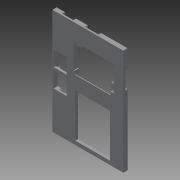
# Autodesk Inventor part: DisplayTop
Saved by Autodesk Inventor 2014 SP1 (Build 180222100, 222)
## iProperties
Created: 2014-03-24
Part Number: DisplayTop
Material: Generic
Document SubType Name: Modeling
Designer: patrigg
Density: 1 g/cm^3
Appearance: Default
Author: patrigg
Autodesk Inventor part; units mm, degrees
ref_plane "YZ Plane" through (0, 0, 0) normal (1, 0, 0) x (0, 1, 0)
ref_plane "XZ Plane" through (0, 0, 0) normal (0, 1, 0) x (-1, 0, 0)
ref_plane "XY Plane" through (0, 0, 0) normal (0, 0, 1) x (1, 0, 0)
sketch "Sketch2" plane through (0, 0, 0) normal (0, 1, 0) x (-1, 0, 0)
  line L0 (-33.5, -50) -> (33.5, -50)
  line L1 (33.5, -50) -> (33.5, 50)
  line L2 (33.5, 50) -> (-33.5, 50)
  line L3 (-33.5, 50) -> (-33.5, -50)
  line L4 (-33.5, -50) -> (33.5, 50) construction
  line L5 (33.5, -50) -> (-33.5, 50) construction
  point P0 (0, 0)
  dimension "d0" = 67
  dimension "d1" = 100
  constraints: 12 end point, 2 midpoint, 2 parallel, 1 horizontal, 1 perpendicular
  measures "d0" distance of L2.end L1.end
  measures "d1" distance of L1.end L0.end
extrude "Extrusion1" add sketch "Sketch2" along normal blind 4
sketch "Sketch3" plane through (0, 4, 0) normal (0, 1, 0) x (1, 0, 0)
  line L0 (33.5, 50) -> (-33.5, 50) projected
  line L1 (-14.5, -4.5) -> (23.5, -4.5)
  line L2 (23.5, -4.5) -> (23.5, 48)
  line L3 (23.5, 48) -> (-14.5, 48)
  line L4 (-14.5, 48) -> (-14.5, -4.5)
  line L5 (-14.5, -4.5) -> (23.5, 48) construction
  line L6 (23.5, -4.5) -> (-14.5, 48) construction
  line L7 (33.5, -50) -> (33.5, 50) projected
  point P0 (0, 0)
  point P1 (4.5, 21.75)
  dimension "d4" = 38
  dimension "d5" = 52.5
  dimension "d6" = 2
  dimension "d99" = 10
  constraints: 12 end point, 2 midpoint, 2 parallel, 1 horizontal, 1 perpendicular
  measures "d4" distance of L3.end L2.end
  measures "d5" distance of L2.end L1.end
  measures "d6" distance between parallel lines of L0 L3
  measures "d99" distance between parallel lines of L7 L2
extrude "Extrusion2" cut sketch "Sketch3" against normal blind 1.5
sketch "Sketch4" plane through (0, 2.5, 0) normal (0, 1, 0) x (1, 0, 0)
  line L0 (23.5, -4.5) -> (-14.5, -4.5) projected
  line L1 (23.5, 48) -> (23.5, -4.5) projected
  line L2 (-14.5, 48) -> (23.5, 48) projected
  line L3 (-14.5, -4.5) -> (-14.5, 48) projected
  line L4 (-12, 46.5) -> (21, 46.5)
  line L5 (21, 46.5) -> (21, 5.5)
  line L6 (21, 5.5) -> (-12, 5.5)
  line L7 (-12, 5.5) -> (-12, 46.5)
  line L8 (-12, 46.5) -> (21, 5.5) construction
  line L9 (21, 46.5) -> (-12, 5.5) construction
  point P0 (0, 0)
  point P1 (4.5, 26)
  dimension "d9" = 10
  dimension "d10" = 1.5
  dimension "d11" = 2.5
  dimension "d12" = 2.5
  constraints: 12 end point, 2 midpoint, 2 parallel, 1 horizontal, 1 perpendicular
  measures "d9" distance between parallel lines of L0 L6
  measures "d10" distance between parallel lines of L2 L4
  measures "d11" distance between parallel lines of L1 L5
  measures "d12" distance between parallel lines of L3 L7
extrude "Extrusion3" cut sketch "Sketch4" against normal blind 2.5 contours L4 L5 L6 L7
sketch "Sketch5" plane through (0, 4, 0) normal (0, 1, 0) x (1, 0, 0)
  line L0 (23.5, 48) -> (23.5, -4.5) projected
  line L1 (23.5, -4.5) -> (-14.5, -4.5) projected
  line L2 (-14.5, -4.5) -> (-14.5, 48) projected
  line L3 (-12.5, -10.5) -> (-12.5, -4.5)
  line L4 (21.5, -10.5) -> (21.5, -4.5)
  line L5 (33.5, 50) -> (-33.5, 50) projected
  line L6 (-12.5, -10.5) -> (21.5, -10.5)
  point P0 (0, 0)
  dimension "d18" = 2
  dimension "d19" = 2
  dimension "d158" = 6
  constraints: 6 end point, 2 perpendicular, 2 point on line, 1 parallel
  measures "d18" distance between parallel lines of L3 L2
  measures "d19" distance between parallel lines of L0 L4
  measures "d158" distance between parallel lines of L1 L6
extrude "Extrusion4" cut sketch "Sketch5" against normal blind 0.25
sketch "Sketch12" plane through (0, 4, 0) normal (0, 1, 0) x (1, 0, 0)
  line L0 (21.5, -10.5) -> (-12.5, -10.5) projected
  line L1 (-13.5, -34.5) -> (24.5, -34.5)
  line L2 (24.5, -34.5) -> (24.5, -10.5)
  line L3 (24.5, -10.5) -> (-13.5, -10.5)
  line L4 (-13.5, -10.5) -> (-13.5, -34.5)
  line L5 (-13.5, -34.5) -> (24.5, -10.5) construction
  line L6 (24.5, -34.5) -> (-13.5, -10.5) construction
  line L7 (23.5, 48) -> (23.5, -4.5) projected
  point P0 (0, 0)
  point P1 (5.5, -22.5)
  point P2 (5.5, -22.5)
  dimension "d120" = 2
  dimension "d121" = 0
  dimension "d58" = 38
  dimension "d59" = 24
  dimension "d100" = 1
  constraints: 12 end point, 3 midpoint, 2 parallel, 1 collinear, 1 horizontal, 1 perpendicular
  measures "d58" distance of L3.end L2.end
  measures "d59" distance of L2.end L1.end
  measures "d100" distance between parallel lines of L2 L7
extrude "Extrusion10" cut sketch "Sketch12" against normal blind 4
sketch "Sketch13" plane through (24.5, 4, 10.5) normal (-1, 0, 0) x (0, 0, 1)
  line L0 (0, 0) -> (24, 0) projected
  line L1 (0, 0) -> (0, -4) projected
  line L2 (24, -4) -> (0, -4) projected
  line L3 (6, 0) -> (6, -4)
  line L4 (0, -2.2) -> (6, -2.2)
  point P0 (-10.5, -4)
  dimension "d67" = 6
  dimension "d74" = 1.8
  constraints: 4 end point, 4 point on line, 2 perpendicular
  measures "d67" distance between parallel lines of L3 L1
  measures "d74" distance between parallel lines of L2 L4
sketch "Sketch14" plane through (-13.5, 4, 34.5) normal (1, 0, 0) x (0, 0, -1)
  line L0 (0, 0) -> (24, 0) projected
  line L1 (0, 0) -> (0, -4)
  line L2 (4.0418, -2.2) -> (4.0418, 0)
  line L3 (24, -4) -> (0, -4) projected
  line L4 (0, -2.2) -> (4.0418, -2.2)
  point P0 (34.5, -4)
  point P1 (0, -2)
  dimension "d79" = 1.8
  constraints: 6 end point, 2 perpendicular, 2 point on line, 1 midpoint
  measures "d79" distance between parallel lines of L3 L4
extrude "Extrusion13" add sketch "Sketch13" along normal blind 4 contours L0 L3 L4 L1
extrude "Extrusion14" add sketch "Sketch14" along normal blind 6
sketch "Sketch16" plane through (0, 3.75, 0) normal (0, 1, 0) x (1, 0, 0)
  line L0 (-12.5, -10.5) -> (-12.5, -4.5) projected
  line L1 (20.5, -10.5) -> (-12.5, -10.5) projected
  line L2 (21.5, -10.5) -> (20.5, -10.5) projected
  line L3 (21.5, -4.5) -> (21.5, -10.5) projected
  line L4 (-12.5, -4.5) -> (21.5, -4.5) projected
  point P0 (0, 0)
extrude "Extrusion15" cut sketch "Sketch16" against normal up to next
sketch "Sketch17" plane through (21.5, 4, 4.5) normal (-1, 0, 0) x (0, 0, 1)
  line L0 (0, -1.5) -> (0, -4) projected
  line L1 (6, -4) -> (0, -4) projected
  line L2 (6, -2.2) -> (6, -4) projected
  line L3 (6, 0) -> (6, -2.2) projected
  line L4 (0, -1.5) -> (-1.7339, -1.5) construction
  line L5 (5, -4) -> (7.1842, -4) construction
  line L6 (0, -1.5) -> (5, -4) construction
  arc A0 (2.5, -2.75) -> (0, -1.5) centre (0, -4.625) ccw
  line L7 (0, -1.5) -> (0, 0) projected
  line L8 (2.5, -2.75) -> (3.4375, -4)
  line L9 (2.9125, -4) -> (2.9125, -3.3)
  point P0 (-4.5, -4)
  dimension "d82" = 1
  dimension "d86" = 0.7
  constraints: 10 end point, 4 point on line, 2 parallel, 2 point on circle, 2 tangent, 1 centre point, 1 midpoint, 1 perpendicular
  measures "d82" distance from line of L2 L5.start
  measures "d86" distance of L9.start L9.end
extrude "Extrusion16" add sketch "Sketch17" along normal up to next contours A0 L8 L9 L1 L0
fillet "Fillet5" radius 1 1 edges at (4.5, 0.7, 7.4125)
sketch "Sketch18" plane through (0, 4, 0) normal (0, 1, 0) x (1, 0, 0)
  line L0 (-33.5, 50) -> (-33.5, -50) projected
  line L1 (-32.5, 14) -> (-20, 14)
  line L2 (-20, 14) -> (-20, -18)
  line L3 (-20, -18) -> (-32.5, -18)
  line L4 (-32.5, -18) -> (-32.5, 14)
  line L5 (33.5, 50) -> (-33.5, 50) projected
  point P0 (0, 0)
  dimension "d89" = 1
  dimension "d97" = 12.5
  dimension "d98" = 32
  dimension "d157" = 36
  constraints: 8 end point, 2 parallel, 1 horizontal, 1 perpendicular
  measures "d89" distance between parallel lines of L0 L4
  measures "d97" distance between parallel lines of L2 L4
  measures "d98" distance between parallel lines of L1 L3
  measures "d157" distance between parallel lines of L1 L5
extrude "Extrusion17" cut sketch "Sketch18" against normal up to next
sketch "Sketch19" plane through (-32.5, 4, 18) normal (1, 0, 0) x (0, 0, -1)
  line L0 (32, -4) -> (0, -4) projected
  line L1 (0, 0) -> (0, -4) projected
  line L2 (14.5, -4) -> (17.5, -4)
  line L3 (17.5, -4) -> (17.5, -2)
  line L4 (17.5, -2) -> (14.5, -2)
  line L5 (14.5, -2) -> (14.5, -4)
  line L6 (14.5, -4) -> (17.5, -2) construction
  line L7 (17.5, -4) -> (14.5, -2) construction
  point P0 (16, -3)
  dimension "d106" = 3
  dimension "d107" = 2
  dimension "d108" = 16
  constraints: 12 end point, 2 midpoint, 2 parallel, 1 collinear, 1 horizontal, 1 perpendicular
  measures "d106" distance of L4.end L3.end
  measures "d107" distance of L3.end L2.end
  measures "d108" distance from line of L1 point (16, -3)
extrude "Extrusion18" add sketch "Sketch19" along normal up to next
sketch "Sketch21" plane through (-32.5, 2, 3.5) normal (0, 1, 0) x (1, 0, 0)
  line L0 (0, 3) -> (12.5, 3) projected
  line L1 (0, 0) -> (12.5, 0) projected
  line L2 (4.75, 1) -> (7.75, 1)
  line L3 (7.75, 1) -> (7.75, 3)
  line L4 (7.75, 3) -> (4.75, 3)
  line L5 (4.75, 3) -> (4.75, 1)
  line L6 (4.75, 1) -> (7.75, 3) construction
  line L7 (7.75, 1) -> (4.75, 3) construction
  point P0 (32.5, 3.5)
  point P1 (6.25, 2)
  point P2 (6.25, 2)
  point P3 (6.25, 0)
  dimension "d111" = 3
  dimension "d112" = 2
  constraints: 12 end point, 4 midpoint, 2 parallel, 1 collinear, 1 horizontal, 1 perpendicular, 1 vertical alignment
  measures "d111" distance of L4.end L3.end
  measures "d112" distance of L3.end L2.end
extrude "Extrusion19" cut sketch "Sketch21" against normal blind 0.5
fillet "Fillet6" radius 1 1 edges at (-26.25, 1.5, 0.5)
sketch "Sketch22" plane through (-32.5, 2, 3.5) normal (0, 1, 0) x (1, 0, 0)
  line L0 (0, 0) -> (12.5, 0) projected
  line L1 (12.5, 3) -> (12.5, 0) projected
  circle A0 centre (2.125, 1.5) radius 1.25
  circle A1 centre (10.375, 1.5) radius 1.25
  point P0 (32.5, 3.5)
  point P1 (6.25, 1.5)
  point P2 (6.25, 0)
  point P3 (12.5, 1.5)
  dimension "d116" = 2.5
  dimension "d117" = 2.5
  dimension "d118" = 8.25
  dimension "d119" = 4.125
  constraints: 3 horizontal alignment, 2 centre point, 2 midpoint, 1 vertical alignment
  measures "d116" diameter of A0
  measures "d117" diameter of A1
  measures "d118" distance of A1.centre A0.centre
  measures "d119" distance of A0.centre point (6.25, 1.5)
extrude "Extrusion20" add sketch "Sketch22" along normal blind 2
chamfer "Chamfer3" distance 0.5 angle 45 2 edges at (-31.625, 4, 2) (-23.375, 4, 2)
sketch "Sketch23" plane through (0, 4, 0) normal (0, 1, 0) x (1, 0, 0)
  line L0 (-33.5, 50) -> (-33.5, -50) projected
  line L1 (-33.5, -50) -> (33.5, -50) projected
  line L2 (-25.75, -34) -> (-15.25, -34)
  line L3 (-15.25, -34) -> (-15.25, -50)
  line L4 (-15.25, -50) -> (-25.75, -50)
  line L5 (-25.75, -50) -> (-25.75, -34)
  line L6 (-25.75, -34) -> (-15.25, -50) construction
  line L7 (-15.25, -34) -> (-25.75, -50) construction
  line L8 (21.5, -4.5) -> (21.5, -10.5) projected
  line L9 (-25.5, -34) -> (-25.5, -42)
  line L10 (-25.5, -42) -> (-25.75, -42)
  line L11 (-15.5, -34) -> (-15.5, -42)
  line L12 (-15.5, -42) -> (-15.25, -42)
  point P0 (0, 0)
  point P1 (-20.5, -42)
  dimension "d125" = 10.5
  dimension "d126" = 16
  dimension "d127" = 13
  dimension "d130" = 0.25
  dimension "d131" = 0.25
  dimension "d132" = 8
  constraints: 20 end point, 4 midpoint, 4 perpendicular, 3 parallel, 2 collinear, 2 point on line, 1 horizontal
  measures "d125" distance of L3.end L4.end
  measures "d126" distance of L2.end L3.end
  measures "d127" distance from line of L0 point (-20.5, -42)
  measures "d130" distance between parallel lines of L5 L9
  measures "d131" distance between parallel lines of L3 L11
  measures "d132" distance of L4.end L10.end
extrude "Extrusion22" cut sketch "Sketch23" against normal blind 2.5 contours L5 L10 L9 L2 L11 L12 L3 L1
sketch "Sketch24" plane through (0, 4, 0) normal (0, 1, 0) x (1, 0, 0)
  line L0 (21.5, -10.5) -> (20.5, -10.5) projected
  line L1 (-25.5, -34) -> (-15.5, -34) projected
  line L2 (-32.5, 14) -> (-20, 14) projected
  line L3 (-20, 14) -> (-20, -18) projected
  line L4 (-20, -18) -> (-32.5, -18) projected
  line L5 (-27.5, 14) -> (-27.5, 22.5)
  line L6 (-27.5, 22.5) -> (-16.5, 22.5)
  line L7 (-16.5, 22.5) -> (-16.5, -29.5711)
  line L8 (-25, 14) -> (-25, 20)
  line L9 (-25, 20) -> (-19, 20)
  line L10 (-19, 20) -> (-19, -25)
  line L11 (-19, -25) -> (-23, -29)
  line L12 (-23, -29) -> (-23, -34)
  line L13 (-16.5, -29.5711) -> (-18, -31.0711)
  line L14 (-18, -31.0711) -> (-18, -34)
  point P0 (0, 0)
  point P1 (-26.25, 14)
  point P2 (-26.25, 14)
  point P3 (-20.5, -34)
  point P4 (-20.5, -34)
  dimension "d135" = 2.5
  dimension "d136" = 2.5
  dimension "d137" = 2.5
  dimension "d139" = 1
  dimension "d140" = 6
  dimension "d142" = 1.25
  dimension "d159" = 5
  dimension "d162" = 135
  dimension "d163" = 135
  dimension "d164" = 5
  dimension "d165" = 5
  dimension "d175" = 2.5
  constraints: 20 end point, 5 perpendicular, 4 point on line, 3 midpoint, 3 parallel, 2 coincident, 1 horizontal alignment
  measures "d135" distance between parallel lines of L8 L5
  measures "d136" distance between parallel lines of L6 L9
  measures "d137" distance between parallel lines of L7 L10
  measures "d139" distance between parallel lines of L3 L10
  measures "d140" distance between parallel lines of L2 L9
  measures "d142" distance from line of L5 point (-26.25, 14)
  measures "d159" distance of L12.end L11.end
  measures "d162" angle of L11 L12
  measures "d163" angle of L7 L13
  measures "d164" distance between parallel lines of L14 L12
  measures "d165" distance from line of L7.end L11
  measures "d175" distance of L14.end point (-20.5, -34)
extrude "Extrusion23" cut sketch "Sketch24" against normal blind 2.5
chamfer "Chamfer4" distance 2 angle 45 2 edges at (-27.5, 2.75, -14) (-25, 2.75, -14)
fillet "Fillet8" radius 2 14 edges at (-29.5, 2.75, -14) (-27.5, 2.75, -16) (-25, 2.75, -16) (-23, 2.75, -14) (-23, 2.75, 34) (-18, 2.75, 34) (-23, 2.75, 29) (-19, 2.75, 25) (-18, 2.75, 31.0711) (-16.5, 2.75, 29.5711) (-19, 2.75, -20) (-25, 2.75, -20) (-27.5, 2.75, -22.5) (-16.5, 2.75, -22.5)
sketch "Sketch25" plane through (0, 4, 0) normal (0, 1, 0) x (1, 0, 0)
  line L0 (33.5, -50) -> (33.5, 50) projected
  line L1 (24.5, -16.5) -> (24.5, -34.5) projected
  line L2 (24.5, -34.5) -> (-7.5, -34.5) projected
  line L3 (24.5, -16.5) -> (33.5, -16.5)
  line L4 (24.5, -33) -> (33.5, -33)
  point P0 (0, 0)
  dimension "d150" = 1.5
  constraints: 4 end point, 3 point on line, 1 parallel, 1 perpendicular
  measures "d150" distance between parallel lines of L2 L4
extrude "Extrusion24" cut sketch "Sketch25" against normal blind 2
sketch "Sketch27" plane through (0, 4, 0) normal (0, 1, 0) x (1, 0, 0)
  line L0 (-15.25, -50) -> (33.5, -50) projected
  line L1 (24.5, -33) -> (24.5, -34.5) projected
  line L2 (-4, -42) -> (8.5, -42)
  line L3 (8.5, -42) -> (8.5, -50)
  line L4 (8.5, -50) -> (-4, -50)
  line L5 (-4, -50) -> (-4, -42)
  line L6 (-4, -42) -> (8.5, -50) construction
  line L7 (8.5, -42) -> (-4, -50) construction
  line L8 (-3.75, -36) -> (8.25, -36)
  line L9 (8.25, -36) -> (8.25, -42)
  line L10 (8.25, -42) -> (-3.75, -42)
  line L11 (-3.75, -42) -> (-3.75, -36)
  line L12 (-3.75, -36) -> (8.25, -42) construction
  line L13 (8.25, -36) -> (-3.75, -42) construction
  point P0 (0, 0)
  point P1 (2.25, -46)
  point P2 (2.25, -39)
  point P3 (2.25, -39)
  point P4 (2.25, -46)
  dimension "d166" = 12.5
  dimension "d167" = 8
  dimension "d168" = 12
  dimension "d169" = 6
  dimension "d170" = 16
  constraints: 24 end point, 6 midpoint, 4 parallel, 2 collinear, 2 horizontal, 2 perpendicular, 1 vertical alignment
  measures "d166" distance of L3.end L4.end
  measures "d167" distance of L2.end L3.end
  measures "d168" distance of L9.end L10.end
  measures "d169" distance of L8.end L9.end
  measures "d170" distance between parallel lines of L3 L1
extrude "Extrusion26" cut sketch "Sketch27" against normal blind 2.5
sketch "Sketch28" plane through (0, 4, 0) normal (0, 1, 0) x (1, 0, 0)
  line L0 (24.5, -34.5) -> (-7.5, -34.5) projected
  line L1 (-3.75, -36) -> (8.25, -36) projected
  line L2 (8.25, -42) -> (8.5, -42) projected
  line L3 (-3.75, -36) -> (-3.75, -34.5)
  line L4 (8.25, -36) -> (8.25, -34.5)
  point P0 (0, 0)
  constraints: 4 end point, 2 perpendicular, 2 point on line
extrude "Extrusion27" cut sketch "Sketch28" against normal blind 2
body "Solid1"
